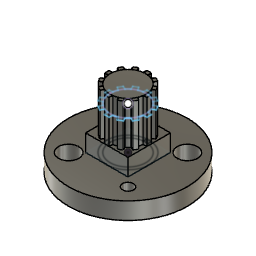
gear_peg_V2 v1 (Autodesk Fusion 360 design; units mm, degrees)
Autodesk Fusion 360 part; units mm, degrees
note: some values were not read from the file. Chosen so that the rebuilt part matches the saved one: which bodies a step acts on; that a step has no effect.
sketch "Sketch1" plane through (0, 0, 0) normal (0, 0, 1) x (1, 0, 0)
  line L0 (12.5, 12.5) -> (-12.5, 12.5)
  line L1 (-12.5, 12.5) -> (-12.5, -12.5)
  line L2 (-12.5, -12.5) -> (12.5, -12.5)
  line L3 (12.5, -12.5) -> (12.5, 12.5)
  line L4 (12.5, 12.5) -> (-12.5, -12.5) construction
  line L5 (-12.5, 12.5) -> (12.5, -12.5) construction
  dimension "d1" = 25
  dimension "d2" = 25
  constraint horizontal L0
  constraint perpendicular L0 L1
  constraint parallel L0 L2
  constraint parallel L1 L3
  constraint coincident L4 origin
  constraint coincident L5 origin
  measures "d1" distance of L1.end L2.end
  measures "d2" distance of L0.end L1.end
extrude "Extrude1" add sketch "Sketch1" against normal blind 10 makes body 1
sketch "Sketch2" plane through (0, 0, -10) normal (0, 0, -1) x (1, 0, 0)
  circle A0 centre (-17.5, 17.5) radius 6
  circle A1 centre (0, 0) radius 35
  circle A2 centre (-17.5, -17.5) radius 3.25
  circle A3 centre (17.5, -17.5) radius 6
  circle A4 centre (17.5, -17.5) radius 3.25
  circle A5 centre (-17.5, 17.5) radius 3.25
  circle A6 centre (17.5, 17.5) radius 3.25
  point P0 (12.5, -14.1834)
  dimension "d6" = 360
  dimension "d7" = 70
  dimension "d8" = 17.5
  dimension "d9" = 17.5
  dimension "d10" = 6.5
  dimension "d11" = 12
  dimension "d12" = 12
  constraint coincident A1.centre origin
  constraint concentric A0 A5
  constraint concentric A3 A4
  constraint coincident P0 A3
  measures "d7" diameter of A1
  measures "d8" vertical distance of A1.centre A6.centre
  measures "d9" horizontal distance of A1.centre A6.centre
  measures "d10" diameter of A6
  measures "d11" diameter of A0
  measures "d12" diameter of A3
extrude "Extrude2" add sketch "Sketch2" along normal blind 10 separate body contours A1 makes body 2
sketch "Sketch3" plane through (0, 0, 0) normal (0, 0, 1) x (-1, 0, 0)
  line L0 (-12.5, 12.5) -> (-12.5, -12.5)
  line L1 (-12.5, -12.5) -> (12.5, -12.5)
  line L2 (12.5, -12.5) -> (12.5, 12.5)
  line L3 (12.5, 12.5) -> (-12.5, 12.5)
  circle A0 centre (0, 0) radius 12.5
  circle A1 centre (0, 0) radius 10.5
  line L4 (0, -12.5) -> (0, -10.5)
  line L5 (1.5, -10.3923) -> (1.25, -12.4373)
  line L6 (-1.25, -12.4373) -> (-1.5, -10.3923)
  line L7 (1.25, -12.4373) -> (1.25, -10.4253)
  line L8 (-1.25, -12.4373) -> (-1.25, -10.4253)
  dimension "d24" = 21
  dimension "d25" = 3
  dimension "d26" = 2.5
  constraint coincident A0.centre A1.centre
  constraint tangent L3 A0
  constraint midpoint L1 L4.start
  constraint coincident A1 L4.end
  constraint perpendicular L1 L4
  constraint coincident A1 L5.start
  constraint coincident A0 L5.end
  constraint coincident A0 L6.start
  constraint coincident A1 L6.end
  constraint symmetric L4 L5 L6
  constraint coincident A1 L7.end
  constraint vertical L7
  constraint coincident A1 L8.end
  constraint parallel L7 L8
  measures "d24" diameter of A1
  measures "d25" horizontal distance of L5.start L6.end
  measures "d26" distance of L5.end L6.start
extrude "Extrude3" add sketch "Sketch3" along normal blind 25 separate body contours A0 A1 L4 L8 | A0 A1 L4 L7 makes body 3
form "Form1" [no effect]
pattern_circular "C-Pattern1" count 12 over 360 about axis through (0, 0, 1.75) along (0, 0, 1) of bodies 3 makes body 4 at (-6.9659, 9.5652, 8.3333) makes body 5 at (-10.8152, 4.8008, 8.3333) makes body 6 at (-11.7667, 1.25, 8.3333) makes body 7 at (-10.8152, -4.8008, 8.3333) makes body 8 at (-6.9659, -9.5652, 8.3333) makes body 9 at (-1.25, -11.7667, 8.3333) makes body 10 at (4.8008, -10.8152, 8.3333) makes body 11 at (9.5652, -6.9659, 8.3333) makes body 12 at (11.7667, -1.25, 8.3333) makes body 13 at (10.8152, 4.8008, 8.3333) makes body 14 at (6.9659, 9.5652, 8.3333)
extrude "Extrude4" add sketch "Sketch3" along normal blind 25 separate body contours A1 makes body 15
sketch "Sketch6" plane through (0, 0, 25) normal (0, 0, 1) x (-1, 0, 0)
  arc A0 (5.1361, -11.3961) -> (7.3012, -10.1461) centre (0, 0) ccw
  line L0 (7.3012, -10.1461) -> (6.4952, -8.25)
  arc A1 (6.4952, -8.25) -> (8.25, -6.4952) centre (0, 0) ccw
  line L1 (8.25, -6.4952) -> (10.1461, -7.3012)
  arc A2 (10.1461, -7.3012) -> (11.3961, -5.1361) centre (0, 0) ccw
  line L2 (11.3961, -5.1361) -> (9.75, -3.8971)
  arc A3 (9.75, -3.8971) -> (10.3923, -1.5) centre (0, 0) ccw
  line L3 (10.3923, -1.5) -> (12.4373, -1.25)
  arc A4 (12.4373, -1.25) -> (12.4373, 1.25) centre (0, 0) ccw
  line L4 (12.4373, 1.25) -> (10.3923, 1.5)
  arc A5 (10.3923, 1.5) -> (9.75, 3.8971) centre (0, 0) ccw
  line L5 (9.75, 3.8971) -> (11.3961, 5.1361)
  arc A6 (11.3961, 5.1361) -> (10.1461, 7.3012) centre (0, 0) ccw
  line L6 (10.1461, 7.3012) -> (8.25, 6.4952)
  arc A7 (8.25, 6.4952) -> (6.4952, 8.25) centre (0, 0) ccw
  line L7 (6.4952, 8.25) -> (7.3012, 10.1461)
  arc A8 (7.3012, 10.1461) -> (5.1361, 11.3961) centre (0, 0) ccw
  line L8 (5.1361, 11.3961) -> (3.8971, 9.75)
  arc A9 (3.8971, 9.75) -> (1.5, 10.3923) centre (0, 0) ccw
  line L9 (1.5, 10.3923) -> (1.25, 12.4373)
  arc A10 (1.25, 12.4373) -> (-1.25, 12.4373) centre (0, 0) ccw
  line L10 (-1.25, 12.4373) -> (-1.5, 10.3923)
  arc A11 (-1.5, 10.3923) -> (-3.8971, 9.75) centre (0, 0) ccw
  line L11 (-3.8971, 9.75) -> (-5.1361, 11.3961)
  arc A12 (-5.1361, 11.3961) -> (-7.3012, 10.1461) centre (0, 0) ccw
  line L12 (-7.3012, 10.1461) -> (-6.4952, 8.25)
  arc A13 (-6.4952, 8.25) -> (-8.25, 6.4952) centre (0, 0) ccw
  line L13 (-8.25, 6.4952) -> (-10.1461, 7.3012)
  arc A14 (-10.1461, 7.3012) -> (-11.3961, 5.1361) centre (0, 0) ccw
  line L14 (-11.3961, 5.1361) -> (-9.75, 3.8971)
  arc A15 (-9.75, 3.8971) -> (-10.3923, 1.5) centre (0, 0) ccw
  line L15 (-10.3923, 1.5) -> (-12.4373, 1.25)
  arc A16 (-12.4373, 1.25) -> (-12.4373, -1.25) centre (0, 0) ccw
  line L16 (-12.4373, -1.25) -> (-10.3923, -1.5)
  arc A17 (-10.3923, -1.5) -> (-9.75, -3.8971) centre (0, 0) ccw
  line L17 (-9.75, -3.8971) -> (-11.3961, -5.1361)
  arc A18 (-11.3961, -5.1361) -> (-10.1461, -7.3012) centre (0, 0) ccw
  line L18 (-10.1461, -7.3012) -> (-8.25, -6.4952)
  arc A19 (-8.25, -6.4952) -> (-6.4952, -8.25) centre (0, 0) ccw
  line L19 (-6.4952, -8.25) -> (-7.3012, -10.1461)
  arc A20 (-7.3012, -10.1461) -> (-5.1361, -11.3961) centre (0, 0) ccw
  line L20 (-5.1361, -11.3961) -> (-3.8971, -9.75)
  arc A21 (-3.8971, -9.75) -> (-1.5, -10.3923) centre (0, 0) ccw
  line L21 (-1.5, -10.3923) -> (-1.25, -12.4373)
  arc A22 (-1.25, -12.4373) -> (1.25, -12.4373) centre (0, 0) ccw
  line L22 (1.25, -12.4373) -> (1.5, -10.3923)
  arc A23 (1.5, -10.3923) -> (3.8971, -9.75) centre (0, 0) ccw
  line L23 (3.8971, -9.75) -> (5.1361, -11.3961)
  circle A24 centre (0, 0) radius 10.5
  constraint concentric A7 A24
extrude "Extrude5" add sketch "Sketch3" along normal blind 25 separate body contours A1 L6 L8 makes body 16
extrude "Extrude6" add sketch "Sketch3" along normal blind 25 separate body contours A1 L5 L7 makes body 17
pattern_circular "C-Pattern2" count 12 over 360 about axis through (0, 0, 1.75) along (0, 0, 1) of bodies 16 17 makes body 18 at (-4.7231, 10.8474, 8.3333) makes body 19 at (-9.514, 7.0325, 8.3333) makes body 20 at (-11.7557, 1.3333, 8.3333) makes body 21 at (-10.8474, -4.7231, 8.3333) makes body 22 at (-7.0325, -9.514, 8.3333) makes body 23 at (-1.3333, -11.7557, 8.3333) makes body 24 at (4.7231, -10.8474, 8.3333) makes body 25 at (9.514, -7.0325, 8.3333) makes body 26 at (11.7557, -1.3333, 8.3333) makes body 27 at (10.8474, 4.7231, 8.3333) makes body 28 at (7.0325, 9.514, 8.3333) makes body 29 at (-6.7639, 8.882, 8.3333) makes body 30 at (-10.2987, 4.3101, 8.3333) makes body 31 at (-11.074, -1.4167, 8.3333) makes body 32 at (-8.882, -6.7639, 8.3333) makes body 33 at (-4.3101, -10.2987, 8.3333) makes body 34 at (1.4167, -11.074, 8.3333) makes body 35 at (6.7639, -8.882, 8.3333) makes body 36 at (10.2987, -4.3101, 8.3333) makes body 37 at (11.074, 1.4167, 8.3333) makes body 38 at (8.882, 6.7639, 8.3333) makes body 39 at (4.3101, 10.2987, 8.3333)
move_body "Move1" bodies 3 17 28 25 21 31 10 13 7 16 19 35 11 39 33 2 30 29 8 38 15 5 14 32 24 6 22 18 23 26 9 12 4 20 27 34 37 36 1 to x (1, 0, 0) y (0, 1, 0) z (0, 0, 1) at (0, 0, 10)
